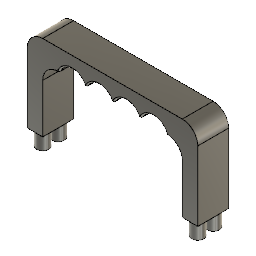
Semana4_Desafio6 (alça) v1 (Autodesk Fusion 360 design; units mm, degrees)
Autodesk Fusion 360 part; units mm, degrees
sketch "Sketch1" plane through (0, 0, 0) normal (0, 1, 0) x (1, 0, 0)
  line L0 (-26.25, -38.343739) -> (-55, -38.343739) construction
  arc A0 (18.397436, -42.203757) -> (34.374038, -41.593739) centre (26.25, -38.343739) ccw
  arc A1 (45, -55) -> (55, -45) centre (45, -45) ccw
  line L1 (34.374038, -41.593739) -> (35, -41.593739)
  arc A2 (0.897436, -42.203757) -> (-0.897436, -42.203757) centre (0, -42.644901) ccw
  arc A3 (18.397436, -42.203757) -> (16.602564, -42.203757) centre (17.5, -42.644901) ccw
  arc A4 (-34.374038, -41.593739) -> (-18.397436, -42.203757) centre (-26.25, -38.343739) ccw
  arc A5 (-55, -45) -> (-45, -55) centre (-45, -45) ccw
  line L2 (-35, -29.593739) -> (35, -29.593739) construction
  line L3 (45, -45) -> (18.125962, -41.593739) construction
  arc A6 (0.897436, -42.203757) -> (16.602564, -42.203757) centre (8.75, -38.343739) ccw
  line L4 (45, -55) -> (-45, -55)
  line L5 (-34.374038, -41.593739) -> (-45, -45) construction
  line L6 (26.25, -38.343739) -> (55, -38.343739) construction
  arc A7 (-45, -31.593739) -> (-35, -41.593739) centre (-35, -31.593739) ccw
  line L7 (0, 0) -> (0, -57.946001) construction
  arc A8 (-16.602564, -42.203757) -> (-18.397436, -42.203757) centre (-17.5, -42.644901) ccw
  arc A9 (-16.602564, -42.203757) -> (-0.897436, -42.203757) centre (-8.75, -38.343739) ccw
  arc A10 (35, -41.593739) -> (45, -31.593739) centre (35, -31.593739) ccw
  line L8 (-35, -41.593739) -> (-34.374038, -41.593739)
  line L9 (-55, -45) -> (-55, 0)
  line L10 (-55, 0) -> (-45, 0)
  line L11 (-45, 0) -> (-45, -31.593739)
  line L12 (55, -45) -> (55, 0)
  line L13 (55, 0) -> (45, 0)
  line L14 (45, 0) -> (45, -31.593739)
  line L15 (55, 0) -> (-55, 0) construction
  dimension "d1" = 10
  dimension "d2" = 10
  dimension "d3" = 10
  dimension "d4" = 17.5
  dimension "d5" = 17.5
  dimension "d6" = 17.5
  dimension "d7" = 17.5
  dimension "d8" = 17.5
  dimension "d9" = 17.5
  dimension "d10" = 17.5
  dimension "d11" = 12
  dimension "d12" = 1
  dimension "d13" = 1
  dimension "d14" = 1
  constraint tangent A5 L4
  constraint tangent A1 L4
  constraint tangent A7 L8
  constraint tangent A10 L8
  constraint equal A7 A10
  constraint coincident A1.centre L3.start
  constraint coincident A5.centre L5.end
  constraint parallel L2 L8
  constraint tangent A4 L2
  constraint tangent A0 L2
  constraint equal L0 L6
  constraint collinear L1 L8
  constraint tangent A4 A8
  constraint tangent A8 A9
  constraint tangent A2 A9
  constraint tangent A2 A6
  constraint tangent A3 A6
  constraint tangent A0 A3
  constraint vertical L7
  constraint tangent A5 L9
  constraint vertical L9
  constraint perpendicular L9 L10
  constraint tangent A7 L11
  constraint tangent A1 L12
  constraint perpendicular L6 L12
  constraint perpendicular L12 L13
  constraint tangent A10 L14
  constraint coincident L7.start origin
  constraint perpendicular L7 L15
  constraint collinear L10 L13
  constraint collinear L10 L15
  measures "d1" radius of A5
  measures "d2" radius of A1
  measures "d3" radius of A7
  measures "d4" diameter of A4
  measures "d5" diameter of A9
  measures "d6" diameter of A6
  measures "d7" diameter of A0
  measures "d11" distance of L2 L8
  measures "d12" radius of A8
  measures "d13" radius of A2
  measures "d14" radius of A3
extrude "Extrude1" add sketch "Sketch1" along normal mid plane 20
fillet "Fillet1" radius 1 14 edges at (-26.583849, -10, 47.087368) (-17.5, -10, 41.644901) (-8.75, -10, 47.093739) (0, -10, 41.644901) (8.75, -10, 47.093739) (17.5, -10, 41.644901) (26.583849, -10, 47.087368) (26.583849, 10, 47.087368) (17.5, 10, 41.644901) (8.75, 10, 47.093739) (0, 10, 41.644901) (-8.75, 10, 47.093739) (-17.5, 10, 41.644901) (-26.583849, 10, 47.087368)
sketch "Sketch2" plane through (0, 0, 0) normal (0, 0, 1) x (1, 0, 0)
  circle A0 centre (-50, -5) radius 4
  circle A1 centre (-50, 5) radius 4
  circle A2 centre (50, -5) radius 4
  circle A3 centre (50, 5) radius 4
  dimension "d18" = 8
  dimension "d19" = 8
  dimension "d20" = 8
  dimension "d21" = 8
  measures "d18" diameter of A0
  measures "d19" diameter of A1
  measures "d20" diameter of A2
  measures "d21" diameter of A3
extrude "Extrude2" add sketch "Sketch2" against normal blind 10
